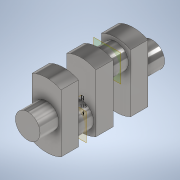
# Autodesk Inventor part: Вал
Saved by Autodesk Inventor 2021 (Build 250183000, 183)
## iProperties
Created: 2020-12-02
Part Number: Вал
Material: Сталь, высокопрочная, низколегированная
Document SubType Name: Modeling
Designer: Тимоха
Mass: 340284 g
Surface Area: 11530.9 cm^2
Volume: 43348.2 cm^3
Density: 7.85 g/cm^3
Appearance: Сталь — полированная
Author: Тимоха
Autodesk Inventor part; units mm, degrees
ref_plane "YZ Plane" through (0, 0, 0) normal (1, 0, 0) x (0, 1, 0)
ref_plane "XZ Plane" through (0, 0, 0) normal (0, 1, 0) x (-1, 0, 0)
sketch "Эскиз1" plane through (0, 0, 0) normal (0, 0, 1) x (1, 0, 0)
  circle A0 centre (0, 0) radius 85
  dimension "d0" = 170
  constraints: 1 centre point, 1 coincident
  measures "d0" diameter of A0
extrude "Выдавливание1" add sketch "Эскиз1" along normal blind 120
sketch "Эскиз2" plane through (0, 0, 0) normal (0, 0, -1) x (-1, 0, 0)
  line L0 (0, 0) -> (0, 115)
  dimension "d3" = 115
  constraints: 2 end point, 1 vertical
  measures "d3" distance of L0.start L0.end
ref_plane "РабПлоскость1" through (0, 0, -120) normal (0, 0, -1) x (-1, 0, 0)
sketch "Эскиз3" plane through (0, 0, -120) normal (0, 0, -1) x (-1, 0, 0)
  line L0 (0, 115) -> (0, 230)
  circle A0 centre (0, 230) radius 85
  point P0 (0, 0)
  dimension "d5" = 115
  dimension "d6" = 170
  constraints: 2 end point, 1 centre point, 1 coincident, 1 vertical
  measures "d5" distance of L0.start L0.end
  measures "d6" diameter of A0
extrude "Выдавливание2" add sketch "Эскиз3" along normal blind 120
sketch "Эскиз4" plane through (0, 0, -120) normal (0, 0, -1) x (-1, 0, 0)
  line L0 (100, -85) -> (100, 315)
  line L1 (100, 315) -> (-100, 315)
  line L2 (-100, 315) -> (-100, -85)
  line L3 (-100, -85) -> (100, -85)
  line L4 (100, -85) -> (-100, 315) construction
  line L5 (100, 315) -> (-100, -85) construction
  arc A0 (100, 315) -> (-100, 315) centre (0, 115) ccw
  arc A1 (-100, -85) -> (100, -85) centre (0, 115) ccw
  point P0 (0, 0)
  dimension "d9" = 400
  dimension "d10" = 200
  constraints: 12 end point, 4 point on circle, 2 centre point, 2 coincident, 2 midpoint, 2 parallel, 1 perpendicular
  measures "d9" distance of L0.start L0.end
  measures "d10" distance of L1.end L0.end
extrude "Выдавливание3" add sketch "Эскиз4" against normal blind 120
ref_plane "РабПлоскость2" through (0, 0, 60) normal (0, 0, 1) x (1, 0, 0)
ref_plane "РабПлоскость3" through (0, 230, -180) normal (0, 0, -1) x (-1, 0, 0)
mirror "Зеркальное отражение1" about plane through (0, 0, 60) normal (0, 0, 1) of "Выдавливание3"
mirror "Зеркальное отражение2" about plane through (0, 230, -180) normal (0, 0, -1) of "Выдавливание3"
sketch "Эскиз5" plane through (0, 115, -360) normal (0, 0, -1) x (-1, 0, 0)
  circle A0 centre (0, 0) radius 85
  point P0 (0, -115)
  dimension "d15" = 170
  constraints: 1 centre point, 1 coincident
  measures "d15" diameter of A0
extrude "Выдавливание4" add sketch "Эскиз5" along normal blind 130
sketch "Эскиз6" plane through (0, 115, 240) normal (0, 0, 1) x (1, 0, 0)
  circle A0 centre (0, 0) radius 85 projected
  point P0 (0, -115)
extrude "Выдавливание5" add sketch "Эскиз6" along normal blind 130
